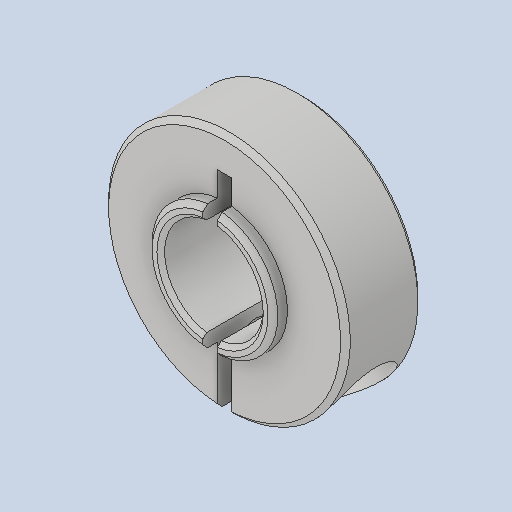
# Autodesk Inventor part: PSCBNJ10-13b
Saved by Autodesk Inventor 2025.1 (Build 291241000, 241)
## iProperties
Category: PARTsolutions
Company: MISUMI
Created: 2024-03-05
Part Number: PSCBNJ10-13b
Material: Generic
Catalog Web Link: www.cadenas.de
Description: SCBNJ, PSCBNJ, SSCBNJ, SCSNAJ, SCSNAWJ, SCLSJ, PSCLSJ, SSCLSJ-b-Set Collars - For Bearing Fixing - Slit Compact Type
Vendor: MISUMI
Document SubType Name: Modeling
Designer: psAdmin
Manufacturer: MISUMI
Mass: 2.97823 g
Surface Area: 20.2401 cm^2
Volume: 2.97823 cm^3
Density: 1 g/cm^3
Appearance: PSOLRGB-191-191-191
PSOL_IDENT_0: {$CADENAS_DATA/23d-libs/misumi/metric/03_set_collars/scbnj_b.prj},237 {VTYP=3D},{NB=PSCBNJ10-13b},{L
PSOL_IDENT_1: INA=PSCBNJ10-13b},{NN=SCBNJ, PSCBNJ, SSCBNJ, SCSNAJ, SCSNAWJ, SCLSJ, PSCLSJ, SSCLSJ-b},{DATE=31.05.2
PSOL_IDENT_2: 023 07:34:13},{GEOMDATE=14.04.2023 07:53:48},{VERSION=},{LINEID=60},{WBVAR=TS,MAT,ST,DSS},{WBNUMERIC=
PSOL_IDENT_3: DSS}  {NB=PSCBNJ10-13b},{LINA=PSCBNJ10-13b},{KT=DUMMY},{PN=PSCBNJ10-13},{TYPE=PSCBNJ},{D=10},{TS=SN}
PSOL_IDENT_4: ,{TS1='SN','Short Nose','LN','Long Nose'},{MAT=1045},{MATA='1045','1045 Carbon Steel','304','304 Sta
PSOL_IDENT_5: inless Steel','2017','2017 Aluminum Alloy'},{ST=Electroless Nickel Plating},{ST0='Black Oxide','Blac
PSOL_IDENT_6: k Oxide','Electroless Nickel Plating','Electroless Nickel Plating'},{DSS=13},{DS1=13,14,16},{AC=Set
PSOL_IDENT_7: Screws 2 Pcs. (SUS) },{AB=6800ZZ(19)},{B=9.5},{B1=12.0},{D1=25},{M=M3},{THMD=3},{BB=8.0},{C=0.5},{L=
PSOL_IDENT_8: 10},{DD=3.5},{R=3.00},{W=1.5},{X=8.0},{Y=4.0},{Z=9.000},{COLOR=0.75,0.75,0.75,0.00}
NB: PSCBNJ10-13b
NN: SCBNJ, PSCBNJ, SSCBNJ, SCSNAJ, SCSNAWJ, SCLSJ, PSCLSJ, SSCLSJ-b
NT: Set Collars - For Bearing Fixing - Slit Compact Type
NBSYN: $PN.b
LINA: PSCBNJ10-13b
CATALOG: Misumi
PN: PSCBNJ10-13
D: 10
TS: Short Nose
MAT: 1045 Carbon Steel
ST: Electroless Nickel Plating
DSS: 13
AC: Set Screws 2 Pcs. (SUS)
AB: 6800ZZ(19)
B: 9.5
B1: 12
D1: 25
M: M3
BB: 8
C: 0.5
L: 10
DD: 3.5
R: 3
W: 1.5
X: 8
Y: 4
Z: 9
SUPPLIER: MISUMI
ARTICLENO: PSCBNJ10-13b
BOMINFO: PSCBNJ10-13b
CREATOR: CADENAS GmbH
Title: PSCBNJ10-13b
Author: Cadenas PARTsolutions
Comments: Set Collars - For Bearing Fixing - Slit Compact Type
Autodesk Inventor part; units mm, degrees
sketch "Sketch_1" plane through (0, 0, 0) normal (1, 0, 0) x (0, 1, 0)
  line L0 (0, -4) -> (0, 5.5)
  line L1 (6, 5.5) -> (5.5, 5.5)
  line L2 (5.5, 5.5) -> (5, 5)
  line L3 (5, 5) -> (5, -3.5)
  line L4 (5, -3.5) -> (5.5, -4)
  line L5 (5.5, -4) -> (12, -4)
  line L6 (12, -4) -> (12.5, -3.5)
  line L7 (12.5, -3.5) -> (12.5, 3.5)
  line L8 (12.5, 3.5) -> (12, 4)
  line L9 (12, 4) -> (6.5, 4)
  line L10 (6.5, 4) -> (6.5, 5)
  line L11 (6.5, 5) -> (6, 5.5)
  constraints: 24 end point
revolve "Revolution1" add sketch "Sketch_1" angle 360 about axis through (0, 0, -4) along (0, 0, -1)
sketch "Sketch_2" plane through (0, 0, 0) normal (0, 0, 1) x (1, 0, 0)
  line L0 (-0.75, -12.5) -> (0.75, -12.5)
  line L1 (0.75, -12.5) -> (0.75, 9)
  line L2 (0.75, 9) -> (-0.75, 9)
  line L3 (-0.75, 9) -> (-0.75, -12.5)
  constraints: 8 end point
extrude "Extrusion1" cut sketch "Sketch_2" along normal mid plane 32
sketch "Sketch_3" plane through (0, 0, 0) normal (0, 0, 1) x (1, 0, 0)
  line L0 (0, -8) -> (12.5, -8)
  line L1 (12.5, -8) -> (12.5, -11)
  line L2 (12.5, -11) -> (4, -11)
  line L3 (4, -11) -> (4, -9.75)
  line L4 (4, -9.75) -> (0, -9.75)
  line L5 (0, -9.75) -> (0, -8)
  line L6 (0, -8) -> (12.5, -8)
  constraints: 14 end point
ref_plane "body_screw_XY" through (4, -8, 0) normal (1, 0, 0) x (0, 0, -1)
ref_plane "body_screw_YZ" through (4, -8, 0) normal (0, 0, -1) x (0, 1, 0)
ref_plane "body_screw_ZX" through (4, -8, 0) normal (0, 1, 0) x (1, 0, 0)
sketch "スケッチ5" plane through (0, 0, -4) normal (0, 0, -1) x (-1, 0, 0)
  circle A0 centre (0, 0) radius 5.1
  dimension "d12" = 10.2
  constraints: 1 centre point, 1 coincident
  measures "d12" diameter of A0
extrude "押し出し2" cut sketch "スケッチ5" against normal through all
ref_plane "作業平面4" through (12.5, 0, 0) normal (1, 0, 0) x (0, 1, 0)
sketch "スケッチ6" plane through (12.5, 0, 0) normal (1, 0, 0) x (0, 1, 0)
  circle A0 centre (-8, 0) radius 1.75 projected
  circle A1 centre (-8, 0) radius 1.7
  circle A2 centre (-8, 0) radius 3.5
  point P0 (0, 0)
  dimension "d15" = 3.4
  dimension "d16" = 7
  constraints: 2 centre point, 2 coincident
  measures "d15" diameter of A1
  measures "d16" diameter of A2
extrude "押し出し3" cut sketch "スケッチ6" against normal through all contours A1
extrude "押し出し4" cut sketch "スケッチ6" against normal blind 8.5 contours A0 | A2
ref_plane "作業平面5" through (-12.5, 0, 0) normal (1, 0, 0) x (0, 1, 0)
extrude "押し出し5" cut sketch "スケッチ6" along normal blind 5 from surface at -25 contours A0 | A2
body "Solid1"
